Autodesk Fusion 360 part; units mm, degrees
(part 4 of 9)
sketch "Sketch5" plane through (0, 0, 11.1324) normal (0, 0, 1) x (-1, 0, 0)
  arc A0 (-57.4236, -34.4162) -> (-57.7889, -35.6603) centre (-49.427, -37.4399) ccw
  arc A1 (-58.3544, -36.0503) -> (-57.7889, -35.6603) centre (-58.278, -35.5562) ccw
  line L0 (-58.3544, -36.0503) -> (-59.6408, -35.8513)
  spline S0 degree 5 poles (-59.6408, -35.8513) (-59.6487, -35.8501) (-59.6643, -35.848) (-59.6879, -35.8455) (-59.7195, -35.8437) (-59.7591, -35.8434) (-59.7989, -35.8445) (-59.8388, -35.8466) (-59.8787, -35.8492) (-59.9187, -35.8521) (-59.9587, -35.8553) (-59.9987, -35.859) (-60.0388, -35.8634) (-60.079, -35.8685) (-60.1191, -35.8743) (-60.1593, -35.8807) (-60.1996, -35.8878) (-60.2398, -35.8953) (-60.2801, -35.9032) (-60.3203, -35.9116) (-60.3606, -35.9203) (-60.4009, -35.9295) (-60.4411, -35.9392) (-60.4814, -35.9493) (-60.5217, -35.9598) (-60.562, -35.9708) (-60.6022, -35.9822) (-60.6425, -35.994) (-60.6827, -36.0062) (-60.723, -36.0188) (-60.7632, -36.0317) (-60.8034, -36.0451) (-60.8435, -36.0588) (-60.8837, -36.0729) (-60.9238, -36.0873) (-60.9639, -36.1021) (-61.004, -36.1173) (-61.044, -36.1329) (-61.084, -36.1487) (-61.124, -36.165) (-61.1639, -36.1816) (-61.2039, -36.1985) (-61.2437, -36.2157) (-61.2836, -36.2333) (-61.3233, -36.2512) (-61.3631, -36.2695) (-61.4028, -36.2881) (-61.4425, -36.307) (-61.4821, -36.3262) (-61.5216, -36.3458) (-61.5611, -36.3656) (-61.6006, -36.3858) (-61.64, -36.4063) (-61.6794, -36.4271) (-61.7187, -36.4482) (-61.7579, -36.4696) (-61.7971, -36.4913) (-61.8362, -36.5134) (-61.8753, -36.5357) (-61.9143, -36.5583) (-61.9532, -36.5812) (-61.9921, -36.6044) (-62.0309, -36.6279) (-62.0696, -36.6517) (-62.1083, -36.6758) (-62.1468, -36.7002) (-62.1854, -36.7249) (-62.2238, -36.7498) (-62.2622, -36.775) (-62.3005, -36.8005) (-62.3387, -36.8263) (-62.3692, -36.8472) (-62.3921, -36.863) (-62.4073, -36.8735) (-62.4149, -36.8788) knots 0 0 0 0 0 0 0.01428571 0.02857143 0.04285714 0.05714286 0.07142857 0.08571429 0.1 0.11428571 0.12857143 0.14285714 0.15714286 0.17142857 0.18571429 0.2 0.21428571 0.22857143 0.24285714 0.25714286 0.27142857 0.28571429 0.3 0.31428571 0.32857143 0.34285714 0.35714286 0.37142857 0.38571429 0.4 0.41428571 0.42857143 0.44285714 0.45714286 0.47142857 0.48571429 0.5 0.51428571 0.52857143 0.54285714 0.55714286 0.57142857 0.58571429 0.6 0.61428571 0.62857143 0.64285714 0.65714286 0.67142857 0.68571429 0.7 0.71428571 0.72857143 0.74285714 0.75714286 0.77142857 0.78571429 0.8 0.81428571 0.82857143 0.84285714 0.85714286 0.87142857 0.88571429 0.9 0.91428571 0.92857143 0.94285714 0.95714286 0.97142857 0.98571429 1 1 1 1 1 1
  arc A2 (-62.4149, -36.8788) -> (-62.4149, -38.001) centre (-49.427, -37.4399) ccw
  spline S1 degree 5 poles (-62.4149, -38.001) (-62.4073, -38.0063) (-62.3921, -38.0168) (-62.3692, -38.0326) (-62.3387, -38.0535) (-62.3005, -38.0792) (-62.2622, -38.1048) (-62.2238, -38.13) (-62.1854, -38.1549) (-62.1468, -38.1796) (-62.1083, -38.204) (-62.0696, -38.2281) (-62.0309, -38.2519) (-61.9921, -38.2754) (-61.9532, -38.2986) (-61.9143, -38.3215) (-61.8753, -38.3441) (-61.8362, -38.3664) (-61.7971, -38.3885) (-61.7579, -38.4102) (-61.7187, -38.4316) (-61.6794, -38.4527) (-61.64, -38.4735) (-61.6006, -38.494) (-61.5611, -38.5142) (-61.5216, -38.534) (-61.4821, -38.5536) (-61.4425, -38.5728) (-61.4028, -38.5917) (-61.3631, -38.6103) (-61.3233, -38.6286) (-61.2836, -38.6465) (-61.2437, -38.6641) (-61.2039, -38.6813) (-61.1639, -38.6982) (-61.124, -38.7148) (-61.084, -38.731) (-61.044, -38.7469) (-61.004, -38.7625) (-60.9639, -38.7777) (-60.9238, -38.7925) (-60.8837, -38.8069) (-60.8435, -38.821) (-60.8034, -38.8347) (-60.7632, -38.848) (-60.723, -38.861) (-60.6827, -38.8736) (-60.6425, -38.8858) (-60.6022, -38.8976) (-60.562, -38.909) (-60.5217, -38.92) (-60.4814, -38.9305) (-60.4411, -38.9406) (-60.4009, -38.9503) (-60.3606, -38.9594) (-60.3203, -38.9682) (-60.2801, -38.9765) (-60.2398, -38.9845) (-60.1996, -38.992) (-60.1593, -38.999) (-60.1191, -39.0055) (-60.079, -39.0113) (-60.0388, -39.0164) (-59.9987, -39.0207) (-59.9587, -39.0245) (-59.9187, -39.0277) (-59.8787, -39.0306) (-59.8388, -39.0332) (-59.7989, -39.0352) (-59.7591, -39.0364) (-59.7195, -39.0361) (-59.6879, -39.0343) (-59.6643, -39.0318) (-59.6487, -39.0297) (-59.6408, -39.0285) knots -1 -1 -1 -1 -1 -1 -0.98571429 -0.97142857 -0.95714286 -0.94285714 -0.92857143 -0.91428571 -0.9 -0.88571429 -0.87142857 -0.85714286 -0.84285714 -0.82857143 -0.81428571 -0.8 -0.78571429 -0.77142857 -0.75714286 -0.74285714 -0.72857143 -0.71428571 -0.7 -0.68571429 -0.67142857 -0.65714286 -0.64285714 -0.62857143 -0.61428571 -0.6 -0.58571429 -0.57142857 -0.55714286 -0.54285714 -0.52857143 -0.51428571 -0.5 -0.48571429 -0.47142857 -0.45714286 -0.44285714 -0.42857143 -0.41428571 -0.4 -0.38571429 -0.37142857 -0.35714286 -0.34285714 -0.32857143 -0.31428571 -0.3 -0.28571429 -0.27142857 -0.25714286 -0.24285714 -0.22857143 -0.21428571 -0.2 -0.18571429 -0.17142857 -0.15714286 -0.14285714 -0.12857143 -0.11428571 -0.1 -0.08571429 -0.07142857 -0.05714286 -0.04285714 -0.02857143 -0.01428571 0 0 0 0 0 0
  line L1 (-59.6408, -39.0285) -> (-58.3544, -38.8295)
  arc A3 (-57.7889, -39.2195) -> (-58.3544, -38.8295) centre (-58.278, -39.3236) ccw
  arc A4 (-57.7889, -39.2195) -> (-57.4236, -40.4636) centre (-49.427, -37.4399) ccw
  arc A5 (-57.6885, -41.0974) -> (-57.4236, -40.4636) centre (-57.8913, -40.6404) ccw
  line L2 (-57.6885, -41.0974) -> (-58.8783, -41.6255)
  spline S2 degree 5 poles (-58.8783, -41.6255) (-58.8855, -41.6287) (-58.8999, -41.6354) (-58.921, -41.6461) (-58.9486, -41.6616) (-58.9821, -41.6828) (-59.0149, -41.7053) (-59.0473, -41.7286) (-59.0795, -41.7523) (-59.1116, -41.7763) (-59.1435, -41.8007) (-59.1752, -41.8255) (-59.2065, -41.8508) (-59.2376, -41.8768) (-59.2682, -41.9034) (-59.2986, -41.9306) (-59.3286, -41.9583) (-59.3584, -41.9863) (-59.388, -42.0148) (-59.4173, -42.0436) (-59.4465, -42.0727) (-59.4754, -42.1022) (-59.504, -42.1321) (-59.5325, -42.1624) (-59.5606, -42.193) (-59.5886, -42.224) (-59.6163, -42.2554) (-59.6438, -42.2871) (-59.671, -42.3191) (-59.6981, -42.3514) (-59.7249, -42.3841) (-59.7515, -42.417) (-59.7779, -42.4503) (-59.804, -42.4838) (-59.83, -42.5177) (-59.8557, -42.5518) (-59.8812, -42.5863) (-59.9065, -42.621) (-59.9316, -42.656) (-59.9564, -42.6912) (-59.9811, -42.7268) (-60.0055, -42.7626) (-60.0297, -42.7987) (-60.0537, -42.835) (-60.0775, -42.8716) (-60.1011, -42.9084) (-60.1244, -42.9455) (-60.1475, -42.9829) (-60.1705, -43.0205) (-60.1932, -43.0583) (-60.2157, -43.0964) (-60.238, -43.1347) (-60.26, -43.1732) (-60.2819, -43.212) (-60.3035, -43.251) (-60.325, -43.2902) (-60.3462, -43.3297) (-60.3672, -43.3694) (-60.388, -43.4093) (-60.4086, -43.4494) (-60.4289, -43.4897) (-60.4491, -43.5302) (-60.469, -43.571) (-60.4887, -43.6119) (-60.5082, -43.6531) (-60.5275, -43.6945) (-60.5466, -43.7361) (-60.5655, -43.7778) (-60.5841, -43.8198) (-60.6025, -43.862) (-60.6207, -43.9043) (-60.6351, -43.9384) (-60.6458, -43.964) (-60.6529, -43.9811) (-60.6564, -43.9897) knots 0 0 0 0 0 0 0.01428571 0.02857143 0.04285714 0.05714286 0.07142857 0.08571429 0.1 0.11428571 0.12857143 0.14285714 0.15714286 0.17142857 0.18571429 0.2 0.21428571 0.22857143 0.24285714 0.25714286 0.27142857 0.28571429 0.3 0.31428571 0.32857143 0.34285714 0.35714286 0.37142857 0.38571429 0.4 0.41428571 0.42857143 0.44285714 0.45714286 0.47142857 0.48571429 0.5 0.51428571 0.52857143 0.54285714 0.55714286 0.57142857 0.58571429 0.6 0.61428571 0.62857143 0.64285714 0.65714286 0.67142857 0.68571429 0.7 0.71428571 0.72857143 0.74285714 0.75714286 0.77142857 0.78571429 0.8 0.81428571 0.82857143 0.84285714 0.85714286 0.87142857 0.88571429 0.9 0.91428571 0.92857143 0.94285714 0.95714286 0.97142857 0.98571429 1 1 1 1 1 1
  arc A6 (-60.6564, -43.9897) -> (-60.0498, -44.9337) centre (-49.427, -37.4399) ccw
  spline S3 degree 5 poles (-60.0498, -44.9337) (-60.0405, -44.934) (-60.022, -44.9347) (-59.9942, -44.9356) (-59.9573, -44.9366) (-59.9112, -44.9377) (-59.8652, -44.9384) (-59.8193, -44.9389) (-59.7734, -44.9391) (-59.7277, -44.939) (-59.6821, -44.9387) (-59.6365, -44.938) (-59.5911, -44.9371) (-59.5457, -44.9359) (-59.5005, -44.9344) (-59.4553, -44.9327) (-59.4103, -44.9306) (-59.3654, -44.9283) (-59.3205, -44.9256) (-59.2758, -44.9227) (-59.2312, -44.9195) (-59.1868, -44.916) (-59.1424, -44.9123) (-59.0982, -44.9082) (-59.0541, -44.9038) (-59.0101, -44.8992) (-58.9663, -44.8942) (-58.9225, -44.889) (-58.879, -44.8835) (-58.8355, -44.8776) (-58.7922, -44.8715) (-58.749, -44.8651) (-58.706, -44.8583) (-58.6632, -44.8513) (-58.6204, -44.844) (-58.5779, -44.8363) (-58.5355, -44.8283) (-58.4932, -44.8201) (-58.4511, -44.8115) (-58.4092, -44.8026) (-58.3675, -44.7934) (-58.3259, -44.7839) (-58.2845, -44.774) (-58.2433, -44.7638) (-58.2023, -44.7533) (-58.1615, -44.7425) (-58.1208, -44.7313) (-58.0804, -44.7198) (-58.0401, -44.708) (-58.0001, -44.6958) (-57.9603, -44.6833) (-57.9207, -44.6704) (-57.8813, -44.6571) (-57.8422, -44.6434) (-57.8034, -44.6294) (-57.7648, -44.615) (-57.7264, -44.6002) (-57.6882, -44.5851) (-57.6503, -44.5697) (-57.6127, -44.5539) (-57.5754, -44.5376) (-57.5384, -44.5207) (-57.5019, -44.5033) (-57.4658, -44.4853) (-57.4301, -44.4668) (-57.3947, -44.4479) (-57.3595, -44.4287) (-57.3245, -44.4093) (-57.2899, -44.3895) (-57.2558, -44.3689) (-57.2226, -44.3473) (-57.197, -44.3287) (-57.1785, -44.3138) (-57.1665, -44.3035) (-57.1606, -44.2983) knots -1 -1 -1 -1 -1 -1 -0.98571429 -0.97142857 -0.95714286 -0.94285714 -0.92857143 -0.91428571 -0.9 -0.88571429 -0.87142857 -0.85714286 -0.84285714 -0.82857143 -0.81428571 -0.8 -0.78571429 -0.77142857 -0.75714286 -0.74285714 -0.72857143 -0.71428571 -0.7 -0.68571429 -0.67142857 -0.65714286 -0.64285714 -0.62857143 -0.61428571 -0.6 -0.58571429 -0.57142857 -0.55714286 -0.54285714 -0.52857143 -0.51428571 -0.5 -0.48571429 -0.47142857 -0.45714286 -0.44285714 -0.42857143 -0.41428571 -0.4 -0.38571429 -0.37142857 -0.35714286 -0.34285714 -0.32857143 -0.31428571 -0.3 -0.28571429 -0.27142857 -0.25714286 -0.24285714 -0.22857143 -0.21428571 -0.2 -0.18571429 -0.17142857 -0.15714286 -0.14285714 -0.12857143 -0.11428571 -0.1 -0.08571429 -0.07142857 -0.05714286 -0.04285714 -0.02857143 -0.01428571 0 0 0 0 0 0
  line L3 (-57.1606, -44.2983) -> (-56.1859, -43.4354)
  arc A7 (-55.4994, -43.4578) -> (-56.1859, -43.4354) centre (-55.8545, -43.8098) ccw
  arc A8 (-55.4994, -43.4578) -> (-54.5195, -44.3069) centre (-49.427, -37.4399) ccw
  arc A9 (-54.3996, -44.9833) -> (-54.5195, -44.3069) centre (-54.8173, -44.7085) ccw
  line L4 (-54.3996, -44.9833) -> (-55.115, -46.0708)
  spline S4 degree 5 poles (-55.115, -46.0708) (-55.1193, -46.0774) (-55.1278, -46.0908) (-55.1399, -46.1112) (-55.1546, -46.1391) (-55.1714, -46.1751) (-55.1868, -46.2118) (-55.2015, -46.2489) (-55.2158, -46.2863) (-55.2298, -46.3238) (-55.2434, -46.3616) (-55.2567, -46.3996) (-55.2693, -46.4378) (-55.2814, -46.4765) (-55.2928, -46.5154) (-55.3036, -46.5547) (-55.3139, -46.5942) (-55.3238, -46.6339) (-55.3333, -46.6738) (-55.3425, -46.7139) (-55.3512, -46.7542) (-55.3596, -46.7946) (-55.3676, -46.8353) (-55.3751, -46.8761) (-55.3822, -46.9171) (-55.389, -46.9583) (-55.3953, -46.9997) (-55.4013, -47.0412) (-55.4069, -47.0829) (-55.4122, -47.1247) (-55.4171, -47.1667) (-55.4217, -47.2088) (-55.4259, -47.251) (-55.4298, -47.2934) (-55.4333, -47.3359) (-55.4365, -47.3785) (-55.4393, -47.4213) (-55.4418, -47.4641) (-55.444, -47.5071) (-55.4458, -47.5502) (-55.4473, -47.5935) (-55.4485, -47.6368) (-55.4494, -47.6802) (-55.4499, -47.7238) (-55.4502, -47.7674) (-55.4501, -47.8111) (-55.4497, -47.855) (-55.4489, -47.8989) (-55.4479, -47.9429) (-55.4466, -47.987) (-55.4449, -48.0312) (-55.4429, -48.0755) (-55.4407, -48.1199) (-55.4381, -48.1643) (-55.4352, -48.2088) (-55.432, -48.2534) (-55.4286, -48.2981) (-55.4248, -48.3428) (-55.4207, -48.3876) (-55.4163, -48.4325) (-55.4116, -48.4774) (-55.4067, -48.5224) (-55.4014, -48.5675) (-55.3959, -48.6126) (-55.39, -48.6578) (-55.3839, -48.703) (-55.3774, -48.7483) (-55.3707, -48.7936) (-55.3637, -48.839) (-55.3564, -48.8844) (-55.3488, -48.9299) (-55.3425, -48.9663) (-55.3377, -48.9937) (-55.3344, -49.0119) (-55.3327, -49.021) knots 0 0 0 0 0 0 0.01428571 0.02857143 0.04285714 0.05714286 0.07142857 0.08571429 0.1 0.11428571 0.12857143 0.14285714 0.15714286 0.17142857 0.18571429 0.2 0.21428571 0.22857143 0.24285714 0.25714286 0.27142857 0.28571429 0.3 0.31428571 0.32857143 0.34285714 0.35714286 0.37142857 0.38571429 0.4 0.41428571 0.42857143 0.44285714 0.45714286 0.47142857 0.48571429 0.5 0.51428571 0.52857143 0.54285714 0.55714286 0.57142857 0.58571429 0.6 0.61428571 0.62857143 0.64285714 0.65714286 0.67142857 0.68571429 0.7 0.71428571 0.72857143 0.74285714 0.75714286 0.77142857 0.78571429 0.8 0.81428571 0.82857143 0.84285714 0.85714286 0.87142857 0.88571429 0.9 0.91428571 0.92857143 0.94285714 0.95714286 0.97142857 0.98571429 1 1 1 1 1 1
  arc A10 (-55.3327, -49.021) -> (-54.312, -49.4872) centre (-49.427, -37.4399) ccw
  spline S5 degree 5 poles (-54.312, -49.4872) (-54.304, -49.4825) (-54.2881, -49.473) (-54.2643, -49.4588) (-54.2326, -49.4397) (-54.1933, -49.4156) (-54.1542, -49.3914) (-54.1153, -49.367) (-54.0766, -49.3423) (-54.0382, -49.3175) (-54, -49.2926) (-53.962, -49.2674) (-53.9243, -49.2421) (-53.8868, -49.2165) (-53.8495, -49.1908) (-53.8125, -49.1649) (-53.7757, -49.1388) (-53.7392, -49.1126) (-53.7029, -49.0862) (-53.6668, -49.0595) (-53.6311, -49.0327) (-53.5955, -49.0058) (-53.5603, -48.9786) (-53.5253, -48.9513) (-53.4905, -48.9238) (-53.456, -48.8961) (-53.4218, -48.8682) (-53.3879, -48.8402) (-53.3542, -48.8119) (-53.3208, -48.7835) (-53.2877, -48.755) (-53.2548, -48.7262) (-53.2223, -48.6973) (-53.19, -48.6682) (-53.1581, -48.6389) (-53.1264, -48.6095) (-53.095, -48.5799) (-53.064, -48.5501) (-53.0332, -48.5201) (-53.0027, -48.4899) (-52.9726, -48.4596) (-52.9428, -48.4291) (-52.9133, -48.3985) (-52.8841, -48.3676) (-52.8553, -48.3366) (-52.8268, -48.3054) (-52.7987, -48.274) (-52.7709, -48.2425) (-52.7434, -48.2108) (-52.7163, -48.1789) (-52.6896, -48.1468) (-52.6632, -48.1146) (-52.6373, -48.0821) (-52.6118, -48.0495) (-52.5868, -48.0167) (-52.5621, -47.9837) (-52.5377, -47.9505) (-52.5138, -47.9172) (-52.4902, -47.8837) (-52.4671, -47.8501) (-52.4445, -47.8162) (-52.4226, -47.782) (-52.4013, -47.7476) (-52.3807, -47.713) (-52.3606, -47.6781) (-52.341, -47.6431) (-52.3218, -47.6079) (-52.3029, -47.5726) (-52.2845, -47.5372) (-52.2669, -47.5015) (-52.2507, -47.4654) (-52.2392, -47.4359) (-52.2317, -47.4134) (-52.2271, -47.3983) (-52.225, -47.3906) knots -1 -1 -1 -1 -1 -1 -0.98571429 -0.97142857 -0.95714286 -0.94285714 -0.92857143 -0.91428571 -0.9 -0.88571429 -0.87142857 -0.85714286 -0.84285714 -0.82857143 -0.81428571 -0.8 -0.78571429 -0.77142857 -0.75714286 -0.74285714 -0.72857143 -0.71428571 -0.7 -0.68571429 -0.67142857 -0.65714286 -0.64285714 -0.62857143 -0.61428571 -0.6 -0.58571429 -0.57142857 -0.55714286 -0.54285714 -0.52857143 -0.51428571 -0.5 -0.48571429 -0.47142857 -0.45714286 -0.44285714 -0.42857143 -0.41428571 -0.4 -0.38571429 -0.37142857 -0.35714286 -0.34285714 -0.32857143 -0.31428571 -0.3 -0.28571429 -0.27142857 -0.25714286 -0.24285714 -0.22857143 -0.21428571 -0.2 -0.18571429 -0.17142857 -0.15714286 -0.14285714 -0.12857143 -0.11428571 -0.1 -0.08571429 -0.07142857 -0.05714286 -0.04285714 -0.02857143 -0.01428571 0 0 0 0 0 0
  line L5 (-52.225, -47.3906) -> (-51.8716, -46.1378)
  arc A11 (-51.2819, -45.7855) -> (-51.8716, -46.1378) centre (-51.3903, -46.2735) ccw
  arc A12 (-51.2819, -45.7855) -> (-49.9985, -45.97) centre (-49.427, -37.4399) ccw
  arc A13 (-49.532, -46.4742) -> (-49.9985, -45.97) centre (-50.0319, -46.4689) ccw
  line L6 (-49.532, -46.4742) -> (-49.5458, -47.7758)
  spline S6 degree 5 poles (-49.5458, -47.7758) (-49.5459, -47.7837) (-49.5458, -47.7996) (-49.5449, -47.8233) (-49.5422, -47.8548) (-49.5369, -47.894) (-49.53, -47.9332) (-49.5223, -47.9724) (-49.5141, -48.0116) (-49.5056, -48.0507) (-49.4967, -48.0899) (-49.4873, -48.129) (-49.4772, -48.1681) (-49.4665, -48.2071) (-49.455, -48.246) (-49.4429, -48.2849) (-49.4302, -48.3237) (-49.4171, -48.3625) (-49.4035, -48.4012) (-49.3895, -48.4398) (-49.3751, -48.4785) (-49.3603, -48.517) (-49.345, -48.5555) (-49.3293, -48.5939) (-49.3131, -48.6323) (-49.2965, -48.6706) (-49.2795, -48.7088) (-49.262, -48.747) (-49.2442, -48.7851) (-49.2261, -48.8231) (-49.2075, -48.8611) (-49.1886, -48.899) (-49.1693, -48.9368) (-49.1497, -48.9745) (-49.1297, -49.0122) (-49.1093, -49.0497) (-49.0885, -49.0872) (-49.0675, -49.1247) (-49.046, -49.162) (-49.0243, -49.1993) (-49.0022, -49.2365) (-48.9798, -49.2735) (-48.957, -49.3106) (-48.9339, -49.3475) (-48.9105, -49.3843) (-48.8868, -49.4211) (-48.8628, -49.4577) (-48.8384, -49.4943) (-48.8137, -49.5307) (-48.7888, -49.5671) (-48.7635, -49.6034) (-48.7379, -49.6396) (-48.712, -49.6757) (-48.6858, -49.7117) (-48.6593, -49.7476) (-48.6325, -49.7834) (-48.6055, -49.819) (-48.5781, -49.8546) (-48.5504, -49.8901) (-48.5225, -49.9255) (-48.4943, -49.9608) (-48.4658, -49.9959) (-48.437, -50.031) (-48.4079, -50.066) (-48.3786, -50.1008) (-48.349, -50.1355) (-48.3191, -50.1702) (-48.2889, -50.2047) (-48.2585, -50.239) (-48.2278, -50.2733) (-48.1968, -50.3075) (-48.1718, -50.3347) (-48.1529, -50.3551) (-48.1403, -50.3687) (-48.134, -50.3754) knots 0 0 0 0 0 0 0.01428571 0.02857143 0.04285714 0.05714286 0.07142857 0.08571429 0.1 0.11428571 0.12857143 0.14285714 0.15714286 0.17142857 0.18571429 0.2 0.21428571 0.22857143 0.24285714 0.25714286 0.27142857 0.28571429 0.3 0.31428571 0.32857143 0.34285714 0.35714286 0.37142857 0.38571429 0.4 0.41428571 0.42857143 0.44285714 0.45714286 0.47142857 0.48571429 0.5 0.51428571 0.52857143 0.54285714 0.55714286 0.57142857 0.58571429 0.6 0.61428571 0.62857143 0.64285714 0.65714286 0.67142857 0.68571429 0.7 0.71428571 0.72857143 0.74285714 0.75714286 0.77142857 0.78571429 0.8 0.81428571 0.82857143 0.84285714 0.85714286 0.87142857 0.88571429 0.9 0.91428571 0.92857143 0.94285714 0.95714286 0.97142857 0.98571429 1 1 1 1 1 1
  arc A14 (-48.134, -50.3754) -> (-47.0233, -50.2157) centre (-49.427, -37.4399) ccw
  spline S7 degree 5 poles (-47.0233, -50.2157) (-47.0191, -50.2075) (-47.0108, -50.1909) (-46.9985, -50.166) (-46.9822, -50.1328) (-46.9621, -50.0913) (-46.9423, -50.0498) (-46.9228, -50.0082) (-46.9035, -49.9666) (-46.8846, -49.925) (-46.866, -49.8833) (-46.8476, -49.8416) (-46.8296, -49.7999) (-46.8119, -49.7581) (-46.7944, -49.7164) (-46.7773, -49.6746) (-46.7604, -49.6328) (-46.7439, -49.5909) (-46.7277, -49.5491) (-46.7117, -49.5072) (-46.6961, -49.4653) (-46.6808, -49.4234) (-46.6658, -49.3815) (-46.6512, -49.3396) (-46.6368, -49.2976) (-46.6228, -49.2557) (-46.609, -49.2138) (-46.5956, -49.1718) (-46.5826, -49.1299) (-46.5698, -49.0879) (-46.5574, -49.046) (-46.5453, -49.0041) (-46.5336, -48.9621) (-46.5222, -48.9202) (-46.5111, -48.8783) (-46.5004, -48.8364) (-46.49, -48.7945) (-46.48, -48.7526) (-46.4703, -48.7108) (-46.461, -48.669) (-46.452, -48.6272) (-46.4434, -48.5854) (-46.4352, -48.5437) (-46.4274, -48.5019) (-46.4199, -48.4603) (-46.4128, -48.4186) (-46.4061, -48.377) (-46.3997, -48.3354) (-46.3938, -48.2939) (-46.3882, -48.2524) (-46.383, -48.211) (-46.3783, -48.1697) (-46.3741, -48.1283) (-46.3703, -48.0871) (-46.3669, -48.0459) (-46.364, -48.0048) (-46.3614, -47.9638) (-46.3593, -47.9228) (-46.3576, -47.8819) (-46.3564, -47.8411) (-46.3557, -47.8004) (-46.3557, -47.7598) (-46.3563, -47.7193) (-46.3577, -47.679) (-46.3597, -47.6389) (-46.3622, -47.5988) (-46.365, -47.5588) (-46.3682, -47.5189) (-46.3718, -47.4792) (-46.3763, -47.4396) (-46.3822, -47.4004) (-46.3885, -47.3694) (-46.3943, -47.3465) (-46.3987, -47.3313) (-46.401, -47.3237) knots -1 -1 -1 -1 -1 -1 -0.98571429 -0.97142857 -0.95714286 -0.94285714 -0.92857143 -0.91428571 -0.9 -0.88571429 -0.87142857 -0.85714286 -0.84285714 -0.82857143 -0.81428571 -0.8 -0.78571429 -0.77142857 -0.75714286 -0.74285714 -0.72857143 -0.71428571 -0.7 -0.68571429 -0.67142857 -0.65714286 -0.64285714 -0.62857143 -0.61428571 -0.6 -0.58571429 -0.57142857 -0.55714286 -0.54285714 -0.52857143 -0.51428571 -0.5 -0.48571429 -0.47142857 -0.45714286 -0.44285714 -0.42857143 -0.41428571 -0.4 -0.38571429 -0.37142857 -0.35714286 -0.34285714 -0.32857143 -0.31428571 -0.3 -0.28571429 -0.27142857 -0.25714286 -0.24285714 -0.22857143 -0.21428571 -0.2 -0.18571429 -0.17142857 -0.15714286 -0.14285714 -0.12857143 -0.11428571 -0.1 -0.08571429 -0.07142857 -0.05714286 -0.04285714 -0.02857143 -0.01428571 0 0 0 0 0 0
  line L7 (-46.401, -47.3237) -> (-46.781, -46.0787)
  arc A15 (-46.4755, -45.4634) -> (-46.781, -46.0787) centre (-46.3028, -45.9327) ccw
  arc A16 (-46.4755, -45.4634) -> (-45.2961, -44.9248) centre (-49.427, -37.4399) ccw
  arc A17 (-44.631, -45.0968) -> (-45.2961, -44.9248) centre (-45.0545, -45.3626) ccw
  line L8 (-44.631, -45.0968) -> (-43.9389, -46.1993)
  spline S8 degree 5 poles (-43.9389, -46.1993) (-43.9347, -46.206) (-43.9261, -46.2192) (-43.9125, -46.2387) (-43.8932, -46.2637) (-43.8675, -46.2939) (-43.8406, -46.3232) (-43.8129, -46.352) (-43.7848, -46.3805) (-43.7564, -46.4088) (-43.7278, -46.4369) (-43.6987, -46.4647) (-43.6692, -46.4922) (-43.6391, -46.5192) (-43.6084, -46.5457) (-43.5772, -46.5719) (-43.5455, -46.5977) (-43.5135, -46.6232) (-43.4811, -46.6484) (-43.4484, -46.6733) (-43.4154, -46.698) (-43.3821, -46.7225) (-43.3485, -46.7466) (-43.3145, -46.7704) (-43.2801, -46.794) (-43.2454, -46.8172) (-43.2104, -46.8401) (-43.1751, -46.8628) (-43.1396, -46.8853) (-43.1037, -46.9074) (-43.0676, -46.9293) (-43.0312, -46.951) (-42.9946, -46.9724) (-42.9576, -46.9935) (-42.9204, -47.0143) (-42.883, -47.0349) (-42.8452, -47.0553) (-42.8073, -47.0754) (-42.7691, -47.0952) (-42.7306, -47.1148) (-42.6919, -47.1341) (-42.653, -47.1532) (-42.6139, -47.172) (-42.5745, -47.1906) (-42.5349, -47.209) (-42.4951, -47.227) (-42.455, -47.2449) (-42.4148, -47.2625) (-42.3743, -47.2798) (-42.3336, -47.2969) (-42.2927, -47.3138) (-42.2516, -47.3304) (-42.2103, -47.3467) (-42.1689, -47.3629) (-42.1272, -47.3787) (-42.0853, -47.3944) (-42.0432, -47.4097) (-42.0009, -47.4249) (-41.9585, -47.4398) (-41.9159, -47.4544) (-41.873, -47.4689) (-41.8301, -47.483) (-41.7869, -47.497) (-41.7435, -47.5107) (-41.7, -47.5241) (-41.6563, -47.5373) (-41.6124, -47.5503) (-41.5684, -47.563) (-41.5242, -47.5755) (-41.4799, -47.5877) (-41.4353, -47.5997) (-41.3996, -47.6091) (-41.3727, -47.616) (-41.3548, -47.6206) (-41.3458, -47.6229) knots 0 0 0 0 0 0 0.01428571 0.02857143 0.04285714 0.05714286 0.07142857 0.08571429 0.1 0.11428571 0.12857143 0.14285714 0.15714286 0.17142857 0.18571429 0.2 0.21428571 0.22857143 0.24285714 0.25714286 0.27142857 0.28571429 0.3 0.31428571 0.32857143 0.34285714 0.35714286 0.37142857 0.38571429 0.4 0.41428571 0.42857143 0.44285714 0.45714286 0.47142857 0.48571429 0.5 0.51428571 0.52857143 0.54285714 0.55714286 0.57142857 0.58571429 0.6 0.61428571 0.62857143 0.64285714 0.65714286 0.67142857 0.68571429 0.7 0.71428571 0.72857143 0.74285714 0.75714286 0.77142857 0.78571429 0.8 0.81428571 0.82857143 0.84285714 0.85714286 0.87142857 0.88571429 0.9 0.91428571 0.92857143 0.94285714 0.95714286 0.97142857 0.98571429 1 1 1 1 1 1
  arc A18 (-41.3458, -47.6229) -> (-40.4977, -46.8881) centre (-49.427, -37.4399) ccw
  spline S9 degree 5 poles (-40.4977, -46.8881) (-40.4987, -46.8788) (-40.5007, -46.8604) (-40.5037, -46.8328) (-40.5079, -46.7961) (-40.5135, -46.7503) (-40.5193, -46.7047) (-40.5253, -46.6592) (-40.5317, -46.6138) (-40.5383, -46.5685) (-40.5451, -46.5234) (-40.5522, -46.4784) (-40.5596, -46.4335) (-40.5673, -46.3888) (-40.5752, -46.3442) (-40.5833, -46.2998) (-40.5918, -46.2555) (-40.6005, -46.2114) (-40.6095, -46.1674) (-40.6187, -46.1236) (-40.6282, -46.0799) (-40.638, -46.0364) (-40.648, -45.993) (-40.6584, -45.9498) (-40.669, -45.9068) (-40.6798, -45.8639) (-40.691, -45.8212) (-40.7024, -45.7787) (-40.714, -45.7363) (-40.726, -45.6941) (-40.7382, -45.6521) (-40.7507, -45.6103) (-40.7635, -45.5687) (-40.7766, -45.5273) (-40.79, -45.486) (-40.8036, -45.445) (-40.8175, -45.4042) (-40.8317, -45.3635) (-40.8462, -45.3231) (-40.8609, -45.2829) (-40.876, -45.2428) (-40.8913, -45.203) (-40.907, -45.1635) (-40.9229, -45.1241) (-40.9392, -45.085) (-40.9557, -45.0462) (-40.9726, -45.0075) (-40.9897, -44.9691) (-41.0071, -44.931) (-41.0249, -44.8931) (-41.043, -44.8555) (-41.0614, -44.8181) (-41.0801, -44.7811) (-41.0992, -44.7443) (-41.1186, -44.7079) (-41.1384, -44.6717) (-41.1584, -44.6358) (-41.1788, -44.6002) (-41.1995, -44.5648) (-41.2205, -44.5298) (-41.2419, -44.4952) (-41.2639, -44.461) (-41.2863, -44.4274) (-41.3093, -44.3942) (-41.3327, -44.3615) (-41.3564, -44.3291) (-41.3804, -44.297) (-41.4046, -44.2652) (-41.4292, -44.2337) (-41.4544, -44.2029) (-41.4805, -44.1731) (-41.5026, -44.1504) (-41.5199, -44.1342) (-41.5318, -44.1238) (-41.5378, -44.1187) knots -1 -1 -1 -1 -1 -1 -0.98571429 -0.97142857 -0.95714286 -0.94285714 -0.92857143 -0.91428571 -0.9 -0.88571429 -0.87142857 -0.85714286 -0.84285714 -0.82857143 -0.81428571 -0.8 -0.78571429 -0.77142857 -0.75714286 -0.74285714 -0.72857143 -0.71428571 -0.7 -0.68571429 -0.67142857 -0.65714286 -0.64285714 -0.62857143 -0.61428571 -0.6 -0.58571429 -0.57142857 -0.55714286 -0.54285714 -0.52857143 -0.51428571 -0.5 -0.48571429 -0.47142857 -0.45714286 -0.44285714 -0.42857143 -0.41428571 -0.4 -0.38571429 -0.37142857 -0.35714286 -0.34285714 -0.32857143 -0.31428571 -0.3 -0.28571429 -0.27142857 -0.25714286 -0.24285714 -0.22857143 -0.21428571 -0.2 -0.18571429 -0.17142857 -0.15714286 -0.14285714 -0.12857143 -0.11428571 -0.1 -0.08571429 -0.07142857 -0.05714286 -0.04285714 -0.02857143 -0.01428571 0 0 0 0 0 0
  line L9 (-41.5378, -44.1187) -> (-42.5306, -43.2768)
  arc A19 (-42.6061, -42.594) -> (-42.5306, -43.2768) centre (-42.2072, -42.8954) ccw
  arc A20 (-42.6061, -42.594) -> (-41.9052, -41.5033) centre (-49.427, -37.4399) ccw
  arc A21 (-41.2527, -41.2883) -> (-41.9052, -41.5033) centre (-41.4653, -41.7409) ccw
  line L10 (-41.2527, -41.2883) -> (-40.0745, -41.8417)
  spline S10 degree 5 poles (-40.0745, -41.8417) (-40.0673, -41.845) (-40.0529, -41.8515) (-40.0309, -41.8606) (-40.0012, -41.8712) (-39.9632, -41.8826) (-39.9247, -41.8927) (-39.8859, -41.902) (-39.8469, -41.9108) (-39.8077, -41.9193) (-39.7684, -41.9274) (-39.7289, -41.9351) (-39.6892, -41.9422) (-39.6493, -41.9487) (-39.6091, -41.9544) (-39.5687, -41.9595) (-39.5281, -41.9641) (-39.4874, -41.9682) (-39.4465, -41.972) (-39.4055, -41.9753) (-39.3644, -41.9782) (-39.3232, -41.9808) (-39.2818, -41.9829) (-39.2403, -41.9845) (-39.1987, -41.9858) (-39.157, -41.9866) (-39.1151, -41.987) (-39.0732, -41.987) (-39.0311, -41.9866) (-38.989, -41.9859) (-38.9468, -41.9848) (-38.9044, -41.9833) (-38.862, -41.9815) (-38.8196, -41.9793) (-38.777, -41.9767) (-38.7343, -41.9738) (-38.6916, -41.9705) (-38.6488, -41.9669) (-38.6059, -41.9629) (-38.563, -41.9586) (-38.52, -41.9539) (-38.477, -41.949) (-38.4338, -41.9436) (-38.3907, -41.938) (-38.3474, -41.932) (-38.3042, -41.9257) (-38.2608, -41.919) (-38.2174, -41.9121) (-38.174, -41.9048) (-38.1306, -41.8972) (-38.0871, -41.8892) (-38.0435, -41.881) (-37.9999, -41.8724) (-37.9563, -41.8636) (-37.9126, -41.8544) (-37.869, -41.8449) (-37.8253, -41.8351) (-37.7815, -41.825) (-37.7377, -41.8146) (-37.694, -41.8038) (-37.6501, -41.7928) (-37.6063, -41.7815) (-37.5625, -41.7699) (-37.5186, -41.758) (-37.4747, -41.7457) (-37.4308, -41.7332) (-37.3869, -41.7204) (-37.343, -41.7073) (-37.2991, -41.6939) (-37.2551, -41.6802) (-37.2112, -41.6662) (-37.176, -41.6548) (-37.1497, -41.6461) (-37.1321, -41.6403) (-37.1233, -41.6373) knots 0 0 0 0 0 0 0.01428571 0.02857143 0.04285714 0.05714286 0.07142857 0.08571429 0.1 0.11428571 0.12857143 0.14285714 0.15714286 0.17142857 0.18571429 0.2 0.21428571 0.22857143 0.24285714 0.25714286 0.27142857 0.28571429 0.3 0.31428571 0.32857143 0.34285714 0.35714286 0.37142857 0.38571429 0.4 0.41428571 0.42857143 0.44285714 0.45714286 0.47142857 0.48571429 0.5 0.51428571 0.52857143 0.54285714 0.55714286 0.57142857 0.58571429 0.6 0.61428571 0.62857143 0.64285714 0.65714286 0.67142857 0.68571429 0.7 0.71428571 0.72857143 0.74285714 0.75714286 0.77142857 0.78571429 0.8 0.81428571 0.82857143 0.84285714 0.85714286 0.87142857 0.88571429 0.9 0.91428571 0.92857143 0.94285714 0.95714286 0.97142857 0.98571429 1 1 1 1 1 1
  arc A22 (-37.1233, -41.6373) -> (-36.8071, -40.5607) centre (-49.427, -37.4399) ccw
  spline S11 degree 5 poles (-36.8071, -40.5607) (-36.813, -40.5534) (-36.8246, -40.539) (-36.8421, -40.5174) (-36.8655, -40.4888) (-36.8949, -40.4533) (-36.9244, -40.4181) (-36.9541, -40.383) (-36.984, -40.3483) (-37.014, -40.3138) (-37.0442, -40.2795) (-37.0745, -40.2455) (-37.1049, -40.2117) (-37.1356, -40.1783) (-37.1663, -40.145) (-37.1972, -40.1121) (-37.2283, -40.0794) (-37.2594, -40.047) (-37.2908, -40.0148) (-37.3222, -39.9829) (-37.3539, -39.9513) (-37.3856, -39.92) (-37.4175, -39.889) (-37.4496, -39.8582) (-37.4817, -39.8277) (-37.514, -39.7975) (-37.5465, -39.7676) (-37.5791, -39.738) (-37.6118, -39.7087) (-37.6447, -39.6797) (-37.6777, -39.651) (-37.7108, -39.6226) (-37.7441, -39.5945) (-37.7774, -39.5667) (-37.811, -39.5392) (-37.8446, -39.512) (-37.8784, -39.4852) (-37.9123, -39.4587) (-37.9464, -39.4325) (-37.9805, -39.4066) (-38.0148, -39.3811) (-38.0493, -39.356) (-38.0838, -39.3311) (-38.1185, -39.3067) (-38.1533, -39.2825) (-38.1883, -39.2588) (-38.2233, -39.2354) (-38.2585, -39.2124) (-38.2938, -39.1897) (-38.3292, -39.1674) (-38.3647, -39.1455) (-38.4004, -39.124) (-38.4362, -39.103) (-38.4721, -39.0824) (-38.5082, -39.0622) (-38.5444, -39.0425) (-38.5807, -39.0231) (-38.617, -39.0042) (-38.6535, -38.9856) (-38.6902, -38.9675) (-38.7269, -38.95) (-38.7638, -38.9331) (-38.8009, -38.917) (-38.8381, -38.9015) (-38.8755, -38.8866) (-38.913, -38.8722) (-38.9505, -38.8582) (-38.9881, -38.8445) (-39.0258, -38.8313) (-39.0636, -38.8189) (-39.1017, -38.808) (-39.1325, -38.8009) (-39.1559, -38.7966) (-39.1715, -38.7943) (-39.1794, -38.7932) knots -1 -1 -1 -1 -1 -1 -0.98571429 -0.97142857 -0.95714286 -0.94285714 -0.92857143 -0.91428571 -0.9 -0.88571429 -0.87142857 -0.85714286 -0.84285714 -0.82857143 -0.81428571 -0.8 -0.78571429 -0.77142857 -0.75714286 -0.74285714 -0.72857143 -0.71428571 -0.7 -0.68571429 -0.67142857 -0.65714286 -0.64285714 -0.62857143 -0.61428571 -0.6 -0.58571429 -0.57142857 -0.55714286 -0.54285714 -0.52857143 -0.51428571 -0.5 -0.48571429 -0.47142857 -0.45714286 -0.44285714 -0.42857143 -0.41428571 -0.4 -0.38571429 -0.37142857 -0.35714286 -0.34285714 -0.32857143 -0.31428571 -0.3 -0.28571429 -0.27142857 -0.25714286 -0.24285714 -0.22857143 -0.21428571 -0.2 -0.18571429 -0.17142857 -0.15714286 -0.14285714 -0.12857143 -0.11428571 -0.1 -0.08571429 -0.07142857 -0.05714286 -0.04285714 -0.02857143 -0.01428571 0 0 0 0 0 0
  line L11 (-39.1794, -38.7932) -> (-40.4697, -38.6217)
  arc A23 (-40.9024, -38.0882) -> (-40.4697, -38.6217) centre (-40.4039, -38.1261) ccw
  arc A24 (-40.9024, -38.0882) -> (-40.9024, -36.7916) centre (-49.427, -37.4399) ccw
  arc A25 (-40.4697, -36.2581) -> (-40.9024, -36.7916) centre (-40.4039, -36.7537) ccw
  line L12 (-40.4697, -36.2581) -> (-39.1794, -36.0865)
  spline S12 degree 5 poles (-39.1794, -36.0865) (-39.1715, -36.0855) (-39.1559, -36.0832) (-39.1325, -36.0789) (-39.1017, -36.0718) (-39.0636, -36.0609) (-39.0258, -36.0485) (-38.9881, -36.0353) (-38.9505, -36.0216) (-38.913, -36.0076) (-38.8755, -35.9932) (-38.8381, -35.9783) (-38.8009, -35.9628) (-38.7638, -35.9467) (-38.7269, -35.9298) (-38.6902, -35.9122) (-38.6535, -35.8942) (-38.617, -35.8756) (-38.5807, -35.8566) (-38.5444, -35.8373) (-38.5082, -35.8175) (-38.4721, -35.7974) (-38.4362, -35.7768) (-38.4004, -35.7558) (-38.3647, -35.7343) (-38.3292, -35.7124) (-38.2938, -35.6901) (-38.2585, -35.6674) (-38.2233, -35.6444) (-38.1883, -35.621) (-38.1533, -35.5972) (-38.1185, -35.5731) (-38.0838, -35.5487) (-38.0493, -35.5238) (-38.0148, -35.4987) (-37.9805, -35.4731) (-37.9464, -35.4473) (-37.9123, -35.4211) (-37.8784, -35.3946) (-37.8446, -35.3677) (-37.811, -35.3406) (-37.7774, -35.3131) (-37.7441, -35.2853) (-37.7108, -35.2572) (-37.6777, -35.2288) (-37.6447, -35.2001) (-37.6118, -35.1711) (-37.5791, -35.1418) (-37.5465, -35.1122) (-37.514, -35.0823) (-37.4817, -35.0521) (-37.4496, -35.0216) (-37.4175, -34.9908) (-37.3856, -34.9598) (-37.3539, -34.9285) (-37.3222, -34.8969) (-37.2908, -34.865) (-37.2594, -34.8328) (-37.2283, -34.8004) (-37.1972, -34.7677) (-37.1663, -34.7348) (-37.1356, -34.7015) (-37.1049, -34.668) (-37.0745, -34.6343) (-37.0442, -34.6003) (-37.014, -34.566) (-36.984, -34.5315) (-36.9541, -34.4968) (-36.9244, -34.4617) (-36.8949, -34.4265) (-36.8655, -34.391) (-36.8421, -34.3623) (-36.8246, -34.3408) (-36.813, -34.3264) (-36.8071, -34.3191) knots 0 0 0 0 0 0 0.01428571 0.02857143 0.04285714 0.05714286 0.07142857 0.08571429 0.1 0.11428571 0.12857143 0.14285714 0.15714286 0.17142857 0.18571429 0.2 0.21428571 0.22857143 0.24285714 0.25714286 0.27142857 0.28571429 0.3 0.31428571 0.32857143 0.34285714 0.35714286 0.37142857 0.38571429 0.4 0.41428571 0.42857143 0.44285714 0.45714286 0.47142857 0.48571429 0.5 0.51428571 0.52857143 0.54285714 0.55714286 0.57142857 0.58571429 0.6 0.61428571 0.62857143 0.64285714 0.65714286 0.67142857 0.68571429 0.7 0.71428571 0.72857143 0.74285714 0.75714286 0.77142857 0.78571429 0.8 0.81428571 0.82857143 0.84285714 0.85714286 0.87142857 0.88571429 0.9 0.91428571 0.92857143 0.94285714 0.95714286 0.97142857 0.98571429 1 1 1 1 1 1
  arc A26 (-36.8071, -34.3191) -> (-37.1233, -33.2424) centre (-49.427, -37.4399) ccw
  spline S13 degree 5 poles (-37.1233, -33.2424) (-37.1321, -33.2395) (-37.1497, -33.2337) (-37.176, -33.225) (-37.2112, -33.2135) (-37.2551, -33.1996) (-37.2991, -33.1859) (-37.343, -33.1725) (-37.3869, -33.1594) (-37.4308, -33.1466) (-37.4747, -33.1341) (-37.5186, -33.1218) (-37.5625, -33.1099) (-37.6063, -33.0983) (-37.6501, -33.087) (-37.694, -33.0759) (-37.7377, -33.0652) (-37.7815, -33.0548) (-37.8253, -33.0447) (-37.869, -33.0349) (-37.9126, -33.0254) (-37.9563, -33.0162) (-37.9999, -33.0074) (-38.0435, -32.9988) (-38.0871, -32.9906) (-38.1306, -32.9826) (-38.174, -32.975) (-38.2174, -32.9677) (-38.2608, -32.9608) (-38.3042, -32.9541) (-38.3474, -32.9478) (-38.3907, -32.9418) (-38.4338, -32.9362) (-38.477, -32.9308) (-38.52, -32.9258) (-38.563, -32.9212) (-38.6059, -32.9169) (-38.6488, -32.9129) (-38.6916, -32.9093) (-38.7343, -32.906) (-38.777, -32.9031) (-38.8196, -32.9005) (-38.862, -32.8983) (-38.9044, -32.8965) (-38.9468, -32.895) (-38.989, -32.8939) (-39.0311, -32.8932) (-39.0732, -32.8928) (-39.1151, -32.8928) (-39.157, -32.8932) (-39.1987, -32.894) (-39.2403, -32.8953) (-39.2818, -32.8969) (-39.3232, -32.899) (-39.3644, -32.9015) (-39.4055, -32.9045) (-39.4465, -32.9078) (-39.4874, -32.9116) (-39.5281, -32.9157) (-39.5687, -32.9203) (-39.6091, -32.9254) (-39.6493, -32.9311) (-39.6892, -32.9376) (-39.7289, -32.9447) (-39.7684, -32.9524) (-39.8077, -32.9605) (-39.8469, -32.969) (-39.8859, -32.9778) (-39.9247, -32.9871) (-39.9632, -32.9972) (-40.0012, -33.0086) (-40.0309, -33.0192) (-40.0529, -33.0283) (-40.0673, -33.0347) (-40.0745, -33.0381) knots -1 -1 -1 -1 -1 -1 -0.98571429 -0.97142857 -0.95714286 -0.94285714 -0.92857143 -0.91428571 -0.9 -0.88571429 -0.87142857 -0.85714286 -0.84285714 -0.82857143 -0.81428571 -0.8 -0.78571429 -0.77142857 -0.75714286 -0.74285714 -0.72857143 -0.71428571 -0.7 -0.68571429 -0.67142857 -0.65714286 -0.64285714 -0.62857143 -0.61428571 -0.6 -0.58571429 -0.57142857 -0.55714286 -0.54285714 -0.52857143 -0.51428571 -0.5 -0.48571429 -0.47142857 -0.45714286 -0.44285714 -0.42857143 -0.41428571 -0.4 -0.38571429 -0.37142857 -0.35714286 -0.34285714 -0.32857143 -0.31428571 -0.3 -0.28571429 -0.27142857 -0.25714286 -0.24285714 -0.22857143 -0.21428571 -0.2 -0.18571429 -0.17142857 -0.15714286 -0.14285714 -0.12857143 -0.11428571 -0.1 -0.08571429 -0.07142857 -0.05714286 -0.04285714 -0.02857143 -0.01428571 0 0 0 0 0 0
  line L13 (-40.0745, -33.0381) -> (-41.2527, -33.5914)
  arc A27 (-41.9052, -33.3765) -> (-41.2527, -33.5914) centre (-41.4653, -33.1389) ccw
  arc A28 (-41.9052, -33.3765) -> (-42.6061, -32.2858) centre (-49.427, -37.4399) ccw
  arc A29 (-42.5306, -31.603) -> (-42.6061, -32.2858) centre (-42.2072, -31.9844) ccw
  line L14 (-42.5306, -31.603) -> (-41.5378, -30.7611)
  spline S14 degree 5 poles (-41.5378, -30.7611) (-41.5318, -30.756) (-41.5199, -30.7455) (-41.5026, -30.7293) (-41.4805, -30.7067) (-41.4544, -30.6769) (-41.4292, -30.6461) (-41.4046, -30.6146) (-41.3804, -30.5828) (-41.3564, -30.5506) (-41.3327, -30.5183) (-41.3093, -30.4856) (-41.2863, -30.4524) (-41.2639, -30.4187) (-41.2419, -30.3846) (-41.2205, -30.35) (-41.1995, -30.315) (-41.1788, -30.2796) (-41.1584, -30.244) (-41.1384, -30.2081) (-41.1186, -30.1719) (-41.0992, -30.1355) (-41.0801, -30.0987) (-41.0614, -30.0617) (-41.043, -30.0243) (-41.0249, -29.9867) (-41.0071, -29.9488) (-40.9897, -29.9106) (-40.9726, -29.8722) (-40.9557, -29.8336) (-40.9392, -29.7947) (-40.9229, -29.7556) (-40.907, -29.7163) (-40.8913, -29.6767) (-40.876, -29.637) (-40.8609, -29.5969) (-40.8462, -29.5567) (-40.8317, -29.5163) (-40.8175, -29.4756) (-40.8036, -29.4348) (-40.79, -29.3937) (-40.7766, -29.3525) (-40.7635, -29.3111) (-40.7507, -29.2695) (-40.7382, -29.2276) (-40.726, -29.1857) (-40.714, -29.1435) (-40.7024, -29.1011) (-40.691, -29.0586) (-40.6798, -29.0159) (-40.669, -28.973) (-40.6584, -28.93) (-40.648, -28.8868) (-40.638, -28.8434) (-40.6282, -28.7999) (-40.6187, -28.7562) (-40.6095, -28.7124) (-40.6005, -28.6684) (-40.5918, -28.6243) (-40.5833, -28.58) (-40.5752, -28.5356) (-40.5673, -28.491) (-40.5596, -28.4463) (-40.5522, -28.4014) (-40.5451, -28.3564) (-40.5383, -28.3113) (-40.5317, -28.266) (-40.5253, -28.2206) (-40.5193, -28.1751) (-40.5135, -28.1295) (-40.5079, -28.0837) (-40.5037, -28.047) (-40.5007, -28.0194) (-40.4987, -28.0009) (-40.4977, -27.9917) knots 0 0 0 0 0 0 0.01428571 0.02857143 0.04285714 0.05714286 0.07142857 0.08571429 0.1 0.11428571 0.12857143 0.14285714 0.15714286 0.17142857 0.18571429 0.2 0.21428571 0.22857143 0.24285714 0.25714286 0.27142857 0.28571429 0.3 0.31428571 0.32857143 0.34285714 0.35714286 0.37142857 0.38571429 0.4 0.41428571 0.42857143 0.44285714 0.45714286 0.47142857 0.48571429 0.5 0.51428571 0.52857143 0.54285714 0.55714286 0.57142857 0.58571429 0.6 0.61428571 0.62857143 0.64285714 0.65714286 0.67142857 0.68571429 0.7 0.71428571 0.72857143 0.74285714 0.75714286 0.77142857 0.78571429 0.8 0.81428571 0.82857143 0.84285714 0.85714286 0.87142857 0.88571429 0.9 0.91428571 0.92857143 0.94285714 0.95714286 0.97142857 0.98571429 1 1 1 1 1 1
  arc A30 (-40.4977, -27.9917) -> (-41.3458, -27.2569) centre (-49.427, -37.4399) ccw
  spline S15 degree 5 poles (-41.3458, -27.2569) (-41.3548, -27.2592) (-41.3727, -27.2637) (-41.3996, -27.2707) (-41.4353, -27.2801) (-41.4799, -27.2921) (-41.5242, -27.3043) (-41.5684, -27.3168) (-41.6124, -27.3295) (-41.6563, -27.3425) (-41.7, -27.3557) (-41.7435, -27.3691) (-41.7869, -27.3828) (-41.8301, -27.3968) (-41.873, -27.4109) (-41.9159, -27.4253) (-41.9585, -27.44) (-42.0009, -27.4549) (-42.0432, -27.47) (-42.0853, -27.4854) (-42.1272, -27.5011) (-42.1689, -27.5169) (-42.2103, -27.5331) (-42.2516, -27.5494) (-42.2927, -27.566) (-42.3336, -27.5829) (-42.3743, -27.6) (-42.4148, -27.6173) (-42.455, -27.6349) (-42.4951, -27.6528) (-42.5349, -27.6708) (-42.5745, -27.6892) (-42.6139, -27.7078) (-42.653, -27.7266) (-42.6919, -27.7457) (-42.7306, -27.765) (-42.7691, -27.7846) (-42.8073, -27.8044) (-42.8452, -27.8245) (-42.883, -27.8448) (-42.9204, -27.8654) (-42.9576, -27.8863) (-42.9946, -27.9074) (-43.0312, -27.9288) (-43.0676, -27.9505) (-43.1037, -27.9724) (-43.1396, -27.9945) (-43.1751, -28.017) (-43.2104, -28.0396) (-43.2454, -28.0626) (-43.2801, -28.0858) (-43.3145, -28.1094) (-43.3485, -28.1332) (-43.3821, -28.1573) (-43.4154, -28.1817) (-43.4484, -28.2064) (-43.4811, -28.2314) (-43.5135, -28.2566) (-43.5455, -28.2821) (-43.5772, -28.3079) (-43.6084, -28.3341) (-43.6391, -28.3606) (-43.6692, -28.3876) (-43.6987, -28.4151) (-43.7278, -28.4429) (-43.7564, -28.471) (-43.7848, -28.4993) (-43.8129, -28.5278) (-43.8406, -28.5566) (-43.8675, -28.5859) (-43.8932, -28.6161) (-43.9125, -28.6411) (-43.9261, -28.6605) (-43.9347, -28.6738) (-43.9389, -28.6805) knots -1 -1 -1 -1 -1 -1 -0.98571429 -0.97142857 -0.95714286 -0.94285714 -0.92857143 -0.91428571 -0.9 -0.88571429 -0.87142857 -0.85714286 -0.84285714 -0.82857143 -0.81428571 -0.8 -0.78571429 -0.77142857 -0.75714286 -0.74285714 -0.72857143 -0.71428571 -0.7 -0.68571429 -0.67142857 -0.65714286 -0.64285714 -0.62857143 -0.61428571 -0.6 -0.58571429 -0.57142857 -0.55714286 -0.54285714 -0.52857143 -0.51428571 -0.5 -0.48571429 -0.47142857 -0.45714286 -0.44285714 -0.42857143 -0.41428571 -0.4 -0.38571429 -0.37142857 -0.35714286 -0.34285714 -0.32857143 -0.31428571 -0.3 -0.28571429 -0.27142857 -0.25714286 -0.24285714 -0.22857143 -0.21428571 -0.2 -0.18571429 -0.17142857 -0.15714286 -0.14285714 -0.12857143 -0.11428571 -0.1 -0.08571429 -0.07142857 -0.05714286 -0.04285714 -0.02857143 -0.01428571 0 0 0 0 0 0
  line L15 (-43.9389, -28.6805) -> (-44.631, -29.783)
  arc A31 (-45.2961, -29.955) -> (-44.631, -29.783) centre (-45.0545, -29.5172) ccw
  arc A32 (-45.2961, -29.955) -> (-46.4755, -29.4164) centre (-49.427, -37.4399) ccw
  arc A33 (-46.781, -28.8011) -> (-46.4755, -29.4164) centre (-46.3028, -28.9471) ccw
  line L16 (-46.781, -28.8011) -> (-46.401, -27.5561)
  spline S16 degree 5 poles (-46.401, -27.5561) (-46.3987, -27.5485) (-46.3943, -27.5333) (-46.3885, -27.5103) (-46.3822, -27.4794) (-46.3763, -27.4402) (-46.3718, -27.4006) (-46.3682, -27.3609) (-46.365, -27.321) (-46.3622, -27.281) (-46.3597, -27.2409) (-46.3577, -27.2008) (-46.3563, -27.1605) (-46.3557, -27.12) (-46.3557, -27.0794) (-46.3564, -27.0387) (-46.3576, -26.9979) (-46.3593, -26.957) (-46.3614, -26.916) (-46.364, -26.875) (-46.3669, -26.8338) (-46.3703, -26.7927) (-46.3741, -26.7514) (-46.3783, -26.7101) (-46.383, -26.6688) (-46.3882, -26.6273) (-46.3938, -26.5859) (-46.3997, -26.5443) (-46.4061, -26.5028) (-46.4128, -26.4612) (-46.4199, -26.4195) (-46.4274, -26.3778) (-46.4352, -26.3361) (-46.4434, -26.2944) (-46.452, -26.2526) (-46.461, -26.2108) (-46.4703, -26.169) (-46.48, -26.1271) (-46.49, -26.0853) (-46.5004, -26.0434) (-46.5111, -26.0015) (-46.5222, -25.9596) (-46.5336, -25.9177) (-46.5453, -25.8757) (-46.5574, -25.8338) (-46.5698, -25.7919) (-46.5826, -25.7499) (-46.5956, -25.708) (-46.609, -25.666) (-46.6228, -25.6241) (-46.6368, -25.5822) (-46.6512, -25.5402) (-46.6658, -25.4983) (-46.6808, -25.4564) (-46.6961, -25.4145) (-46.7117, -25.3726) (-46.7277, -25.3307) (-46.7439, -25.2889) (-46.7604, -25.247) (-46.7773, -25.2052) (-46.7944, -25.1634) (-46.8119, -25.1216) (-46.8296, -25.0799) (-46.8476, -25.0382) (-46.866, -24.9965) (-46.8846, -24.9548) (-46.9035, -24.9132) (-46.9228, -24.8716) (-46.9423, -24.83) (-46.9621, -24.7884) (-46.9822, -24.7469) (-46.9985, -24.7138) (-47.0108, -24.6889) (-47.0191, -24.6723) (-47.0233, -24.6641) knots 0 0 0 0 0 0 0.01428571 0.02857143 0.04285714 0.05714286 0.07142857 0.08571429 0.1 0.11428571 0.12857143 0.14285714 0.15714286 0.17142857 0.18571429 0.2 0.21428571 0.22857143 0.24285714 0.25714286 0.27142857 0.28571429 0.3 0.31428571 0.32857143 0.34285714 0.35714286 0.37142857 0.38571429 0.4 0.41428571 0.42857143 0.44285714 0.45714286 0.47142857 0.48571429 0.5 0.51428571 0.52857143 0.54285714 0.55714286 0.57142857 0.58571429 0.6 0.61428571 0.62857143 0.64285714 0.65714286 0.67142857 0.68571429 0.7 0.71428571 0.72857143 0.74285714 0.75714286 0.77142857 0.78571429 0.8 0.81428571 0.82857143 0.84285714 0.85714286 0.87142857 0.88571429 0.9 0.91428571 0.92857143 0.94285714 0.95714286 0.97142857 0.98571429 1 1 1 1 1 1
  arc A34 (-47.0233, -24.6641) -> (-48.134, -24.5044) centre (-49.427, -37.4399) ccw
  spline S17 degree 5 poles (-48.134, -24.5044) (-48.1403, -24.5111) (-48.1529, -24.5247) (-48.1718, -24.5451) (-48.1968, -24.5723) (-48.2278, -24.6065) (-48.2585, -24.6407) (-48.2889, -24.6751) (-48.3191, -24.7096) (-48.349, -24.7443) (-48.3786, -24.779) (-48.4079, -24.8138) (-48.437, -24.8488) (-48.4658, -24.8838) (-48.4943, -24.919) (-48.5225, -24.9543) (-48.5504, -24.9897) (-48.5781, -25.0252) (-48.6055, -25.0607) (-48.6325, -25.0964) (-48.6593, -25.1322) (-48.6858, -25.1681) (-48.712, -25.2041) (-48.7379, -25.2402) (-48.7635, -25.2764) (-48.7888, -25.3127) (-48.8137, -25.349) (-48.8384, -25.3855) (-48.8628, -25.4221) (-48.8868, -25.4587) (-48.9105, -25.4955) (-48.9339, -25.5323) (-48.957, -25.5692) (-48.9798, -25.6062) (-49.0022, -25.6433) (-49.0243, -25.6805) (-49.046, -25.7178) (-49.0675, -25.7551) (-49.0885, -25.7925) (-49.1093, -25.83) (-49.1297, -25.8676) (-49.1497, -25.9053) (-49.1693, -25.943) (-49.1886, -25.9808) (-49.2075, -26.0187) (-49.2261, -26.0567) (-49.2442, -26.0947) (-49.262, -26.1328) (-49.2795, -26.171) (-49.2965, -26.2092) (-49.3131, -26.2475) (-49.3293, -26.2859) (-49.345, -26.3243) (-49.3603, -26.3628) (-49.3751, -26.4013) (-49.3895, -26.44) (-49.4035, -26.4786) (-49.4171, -26.5173) (-49.4302, -26.5561) (-49.4429, -26.5949) (-49.455, -26.6338) (-49.4665, -26.6727) (-49.4772, -26.7117) (-49.4873, -26.7508) (-49.4967, -26.7899) (-49.5056, -26.8291) (-49.5141, -26.8682) (-49.5223, -26.9074) (-49.53, -26.9465) (-49.5369, -26.9858) (-49.5422, -27.025) (-49.5449, -27.0565) (-49.5458, -27.0802) (-49.5459, -27.096) (-49.5458, -27.104) knots -1 -1 -1 -1 -1 -1 -0.98571429 -0.97142857 -0.95714286 -0.94285714 -0.92857143 -0.91428571 -0.9 -0.88571429 -0.87142857 -0.85714286 -0.84285714 -0.82857143 -0.81428571 -0.8 -0.78571429 -0.77142857 -0.75714286 -0.74285714 -0.72857143 -0.71428571 -0.7 -0.68571429 -0.67142857 -0.65714286 -0.64285714 -0.62857143 -0.61428571 -0.6 -0.58571429 -0.57142857 -0.55714286 -0.54285714 -0.52857143 -0.51428571 -0.5 -0.48571429 -0.47142857 -0.45714286 -0.44285714 -0.42857143 -0.41428571 -0.4 -0.38571429 -0.37142857 -0.35714286 -0.34285714 -0.32857143 -0.31428571 -0.3 -0.28571429 -0.27142857 -0.25714286 -0.24285714 -0.22857143 -0.21428571 -0.2 -0.18571429 -0.17142857 -0.15714286 -0.14285714 -0.12857143 -0.11428571 -0.1 -0.08571429 -0.07142857 -0.05714286 -0.04285714 -0.02857143 -0.01428571 0 0 0 0 0 0
  line L17 (-49.5458, -27.104) -> (-49.532, -28.4056)
  arc A35 (-49.9985, -28.9098) -> (-49.532, -28.4056) centre (-50.0319, -28.4109) ccw
  arc A36 (-49.9985, -28.9098) -> (-51.2819, -29.0943) centre (-49.427, -37.4399) ccw
  arc A37 (-51.8716, -28.742) -> (-51.2819, -29.0943) centre (-51.3903, -28.6062) ccw
  line L18 (-51.8716, -28.742) -> (-52.225, -27.4892)
  spline S18 degree 5 poles (-52.225, -27.4892) (-52.2271, -27.4815) (-52.2317, -27.4664) (-52.2392, -27.4439) (-52.2507, -27.4144) (-52.2669, -27.3783) (-52.2845, -27.3426) (-52.3029, -27.3072) (-52.3218, -27.2719) (-52.341, -27.2367) (-52.3606, -27.2017) (-52.3807, -27.1668) (-52.4013, -27.1322) (-52.4226, -27.0978) (-52.4445, -27.0636) (-52.4671, -27.0297) (-52.4902, -26.9961) (-52.5138, -26.9626) (-52.5377, -26.9293) (-52.5621, -26.8961) (-52.5868, -26.8631) (-52.6118, -26.8303) (-52.6373, -26.7977) (-52.6632, -26.7652) (-52.6896, -26.733) (-52.7163, -26.7009) (-52.7434, -26.669) (-52.7709, -26.6373) (-52.7987, -26.6058) (-52.8268, -26.5744) (-52.8553, -26.5432) (-52.8841, -26.5122) (-52.9133, -26.4813) (-52.9428, -26.4507) (-52.9726, -26.4202) (-53.0027, -26.3898) (-53.0332, -26.3597) (-53.064, -26.3297) (-53.095, -26.2999) (-53.1264, -26.2703) (-53.1581, -26.2409) (-53.19, -26.2116) (-53.2223, -26.1825) (-53.2548, -26.1536) (-53.2877, -26.1248) (-53.3208, -26.0962) (-53.3542, -26.0678) (-53.3879, -26.0396) (-53.4218, -26.0116) (-53.456, -25.9837) (-53.4905, -25.956) (-53.5253, -25.9285) (-53.5603, -25.9012) (-53.5955, -25.874) (-53.6311, -25.8471) (-53.6668, -25.8203) (-53.7029, -25.7936) (-53.7392, -25.7672) (-53.7757, -25.7409) (-53.8125, -25.7149) (-53.8495, -25.689) (-53.8868, -25.6633) (-53.9243, -25.6377) (-53.962, -25.6124) (-54, -25.5872) (-54.0382, -25.5622) (-54.0766, -25.5374) (-54.1153, -25.5128) (-54.1542, -25.4884) (-54.1933, -25.4642) (-54.2326, -25.4401) (-54.2643, -25.421) (-54.2881, -25.4068) (-54.304, -25.3973) (-54.312, -25.3926) knots 0 0 0 0 0 0 0.01428571 0.02857143 0.04285714 0.05714286 0.07142857 0.08571429 0.1 0.11428571 0.12857143 0.14285714 0.15714286 0.17142857 0.18571429 0.2 0.21428571 0.22857143 0.24285714 0.25714286 0.27142857 0.28571429 0.3 0.31428571 0.32857143 0.34285714 0.35714286 0.37142857 0.38571429 0.4 0.41428571 0.42857143 0.44285714 0.45714286 0.47142857 0.48571429 0.5 0.51428571 0.52857143 0.54285714 0.55714286 0.57142857 0.58571429 0.6 0.61428571 0.62857143 0.64285714 0.65714286 0.67142857 0.68571429 0.7 0.71428571 0.72857143 0.74285714 0.75714286 0.77142857 0.78571429 0.8 0.81428571 0.82857143 0.84285714 0.85714286 0.87142857 0.88571429 0.9 0.91428571 0.92857143 0.94285714 0.95714286 0.97142857 0.98571429 1 1 1 1 1 1
  arc A38 (-54.312, -25.3926) -> (-55.3327, -25.8588) centre (-49.427, -37.4399) ccw